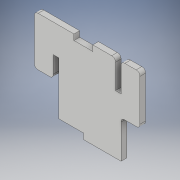
# Autodesk Inventor part: front_right_v2
Saved by Autodesk Inventor 2017.2 (Build 212233000, 233)
## iProperties
Created: 2017-06-09
Part Number: front_right_v2
Material: Generic
Document SubType Name: Modeling
Designer: SandeepSH
Density: 1 g/cm^3
Appearance: Default
Author: SandeepSH
Autodesk Inventor part; units mm, degrees
ref_plane "YZ Plane" through (0, 0, 0) normal (1, 0, 0) x (0, 1, 0)
ref_plane "XZ Plane" through (0, 0, 0) normal (0, 1, 0) x (-1, 0, 0)
ref_plane "XY Plane" through (0, 0, 0) normal (0, 0, 1) x (1, 0, 0)
sketch "Sketch1" plane through (0, 0, 0) normal (0, 0, 1) x (1, 0, 0)
  line L0 (0, 0) -> (36, 0)
  line L1 (36, 0) -> (36, 46)
  line L2 (36, 46) -> (0, 46)
  line L3 (0, 46) -> (0, 0)
  dimension "d0" = 36
  dimension "d1" = 46
  constraints: 8 end point, 2 parallel, 1 horizontal, 1 perpendicular
  measures "d0" distance of L2.end L1.end
  measures "d1" distance of L1.end L0.end
extrude "Extrusion1" add sketch "Sketch1" along normal blind 3
sketch "Sketch2" plane through (0, 0, 3) normal (0, 0, 1) x (1, 0, 0)
  line L0 (0, 0) -> (16, 0)
  line L1 (16, 0) -> (16, 3)
  line L2 (16, 3) -> (0, 3)
  line L3 (0, 3) -> (0, 0)
  line L4 (36, 0) -> (36, 46) projected
  line L5 (0, 3) -> (3, 3)
  line L6 (3, 3) -> (3, 31)
  line L7 (3, 31) -> (0, 31)
  line L8 (0, 31) -> (0, 3)
  line L9 (36, 46) -> (0, 46) projected
  line L10 (11, 46) -> (21, 46)
  line L11 (21, 46) -> (21, 43)
  line L12 (21, 43) -> (11, 43)
  line L13 (11, 43) -> (11, 46)
  line L14 (36, 46) -> (33, 46)
  line L15 (33, 46) -> (33, 31)
  line L16 (33, 31) -> (36, 31)
  line L17 (36, 31) -> (36, 46)
  dimension "d4" = 3
  dimension "d5" = 20
  dimension "d6" = 3
  dimension "d7" = 15
  dimension "d8" = 10
  dimension "d9" = 3
  dimension "d10" = 15
  dimension "d11" = 3
  dimension "d12" = 15
  constraints: 32 end point, 8 parallel, 4 horizontal, 4 perpendicular, 1 point on line
  measures "d4" distance of L1.end L0.end
  measures "d5" distance between parallel lines of L4 L1
  measures "d6" distance of L7.end L6.end
  measures "d7" distance between parallel lines of L9 L7
  measures "d8" distance of L11.end L12.end
  measures "d9" distance of L10.end L11.end
  measures "d10" distance between parallel lines of L4 L11
  measures "d11" distance of L16.end L15.end
  measures "d12" distance of L15.end L14.end
extrude "Extrusion2" cut sketch "Sketch2" against normal through all
sketch "Sketch3" plane through (0, 0, 3) normal (0, 0, 1) x (1, 0, 0)
  line L0 (11, 46) -> (0, 46) projected
  line L1 (0, 46) -> (-10, 46)
  line L2 (-10, 46) -> (-10, 20)
  line L3 (-10, 20) -> (0, 20)
  line L4 (0, 20) -> (0, 46)
  line L5 (16, 0) -> (36, 0) projected
  line L6 (36, 46) -> (46, 46)
  line L7 (46, 46) -> (46, 20)
  line L8 (46, 20) -> (36, 20)
  line L9 (36, 20) -> (36, 46)
  line L10 (33, 46) -> (21, 46) projected
  point P0 (0, 0)
  dimension "d15" = 10
  dimension "d16" = 20
  dimension "d17" = 10
  dimension "d18" = 20
  constraints: 16 end point, 4 parallel, 2 horizontal, 2 perpendicular, 1 collinear
  measures "d15" distance of L3.end L2.end
  measures "d16" distance between parallel lines of L5 L3
  measures "d17" distance of L7.end L8.end
  measures "d18" distance between parallel lines of L5 L8
extrude "Extrusion3" add sketch "Sketch3" against normal blind 3
fillet "Fillet1" radius 2 7 edges at (0, 20, 1.5) (46, 20, 1.5) (46, 46, 1.5) (33, 46, 1.5) (36, 46, 1.5) (36, 20, 1.5) (-10, 20, 1.5) curvature continuous yes
fillet "Fillet2" radius 2 1 edges at (-10, 46, 1.5) curvature continuous yes
body "Solid1"
